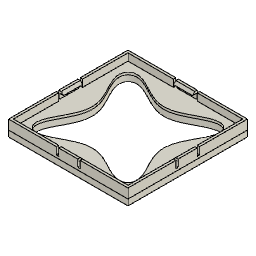
aufsatz (v3) v6 (Autodesk Fusion 360 design; units mm, degrees)
Autodesk Fusion 360 part; units mm, degrees
sketch "Skizze1" plane through (0, 0, 0) normal (0, 0, 1) x (1, 0, 0)
  line L0 (25, -25) -> (-25, -25) construction
  line L1 (-25, -25) -> (-25, 25) construction
  line L2 (-25, 25) -> (25, 25) construction
  line L3 (25, 25) -> (25, -25) construction
  line L4 (25, -25) -> (-25, 25) construction
  line L5 (-25, -25) -> (25, 25) construction
  line L6 (0, 25) -> (0, 20) construction
  line L7 (2.5, 22.5) -> (-2.5, 22.5)
  line L8 (-2.5, 22.5) -> (-2.5, 17.5)
  line L9 (-2.5, 17.5) -> (2.5, 17.5)
  line L10 (2.5, 17.5) -> (2.5, 22.5)
  line L11 (2.5, 22.5) -> (-2.5, 17.5) construction
  line L12 (-2.5, 22.5) -> (2.5, 17.5) construction
  circle A0 centre (0, 20) radius 5 construction
  line L13 (-22.5, -2.5) -> (-17.5, -2.5)
  line L14 (-17.5, -2.5) -> (-17.5, 2.5)
  line L15 (-22.5, 2.5) -> (-22.5, -2.5)
  line L16 (-17.5, 2.5) -> (-22.5, 2.5)
  line L17 (2.5, -22.5) -> (2.5, -17.5)
  line L18 (2.5, -17.5) -> (-2.5, -17.5)
  line L19 (-2.5, -22.5) -> (2.5, -22.5)
  line L20 (-2.5, -17.5) -> (-2.5, -22.5)
  line L21 (22.5, 2.5) -> (17.5, 2.5)
  line L22 (17.5, 2.5) -> (17.5, -2.5)
  line L23 (22.5, -2.5) -> (22.5, 2.5)
  line L24 (17.5, -2.5) -> (22.5, -2.5)
  line L25 (0, 25) -> (0, 15) construction
  line L26 (-25, -25) -> (25, -25)
  line L27 (25, -25) -> (25, 25)
  line L28 (25, 25) -> (-25, 25)
  line L29 (-25, 25) -> (-25, -25)
  spline S0 degree 5 poles (-20.0503, -20.0503) (-19.6556, -20.4489) (-18.686, -21.0653) (-16.7589, -21.3768) (-13.6473, -20.413) (-9.2487, -17.9258) (-4.6595, -15.5152) (0, -14.5056) (4.6595, -15.5149) (9.249, -17.9252) (13.6484, -20.4119) (17.5385, -21.6165) (20.5241, -20.5233) (21.5929, -17.5167) (20.3741, -13.6196) (17.8872, -9.2258) (15.4909, -4.649) (14.5051, -0.0015) (15.5403, 4.6523) (17.9692, 9.2426) (20.4589, 13.6458) (21.6478, 17.539) (20.5227, 20.524) (17.4867, 21.5928) (13.5795, 20.3782) (9.1932, 17.896) (4.6342, 15.5003) (0.0037, 14.5069) (-4.642, 15.5269) (-9.233, 17.9402) (-13.6414, 20.424) (-17.5392, 21.6225) (-20.5241, 20.5233) (-21.5922, 17.5107) (-20.3811, 13.6075) (-17.9032, 9.2107) (-15.5084, 4.637) (-14.5087, 0.0002) (-15.515, -4.6374) (-17.9137, -9.2128) (-20.3911, -13.611) (-21.3564, -16.7334) (-21.0536, -18.6733) (-20.4449, -19.6516) (-20.0503, -20.0503) knots 0 0 0 0 0 0 0.025 0.05 0.075 0.1 0.125 0.15 0.175 0.2 0.225 0.25 0.275 0.3 0.325 0.35 0.375 0.4 0.425 0.45 0.475 0.5 0.525 0.55 0.575 0.6 0.625 0.65 0.675 0.7 0.725 0.75 0.775 0.8 0.825 0.85 0.875 0.9 0.925 0.95 0.975 1 1 1 1 1 1
  line L30 (-15.1005, 25.0697) -> (-25, 15.0308)
  line L31 (25.1278, 15.1005) -> (14.9727, 25)
  line L32 (-25, -15.0497) -> (-15.1005, -25.0508)
  line L33 (15.1005, -25.0545) -> (25, -15.046)
  point P0 (0, 20)
  point P1 (0, -15)
  point P2 (20.0503, -20.0503)
  point P3 (15, 0)
  point P4 (20.0503, 20.0503)
  point P5 (-20.0503, 20.0503)
  point P6 (-15, 0)
  dimension "d1" = 50
  dimension "d2" = 50
  dimension "d3" = 5
  dimension "d4" = 5
  dimension "d5" = 5
  dimension "d7" = 10
  dimension "d14" = 10
  dimension "d19" = 7
  dimension "d20" = 7
  dimension "d21" = 7
  dimension "d22" = 7
  constraint horizontal L0
  constraint perpendicular L0 L1
  constraint parallel L0 L2
  constraint parallel L1 L3
  constraint coincident L4 origin
  constraint coincident L5 origin
  constraint midpoint L2 L6.start
  constraint perpendicular L2 L6
  constraint horizontal L7
  constraint perpendicular L7 L8
  constraint parallel L7 L9
  constraint parallel L8 L10
  constraint coincident L11 P0
  constraint coincident L12 P0
  constraint coincident P0 L6.end
  constraint coincident L6.start L25.start
  constraint parallel L6 L25
  constraint horizontal L26
  constraint vertical L27
  constraint horizontal L28
  constraint vertical L29
  constraint coincident L5 S0.start
  constraint coincident L4 P2
  constraint coincident L5 P4
  constraint coincident L4 P5
  constraint midpoint P5 L30
  constraint coincident L1 L30.end
  constraint midpoint P4 L31
  constraint coincident L28 L31.end
  constraint midpoint S0.start L32
  constraint midpoint P2 L33
  constraint coincident L3 L33.end
  measures "d1" distance of L1.end L2.end
  measures "d2" distance of L0.end L1.end
  measures "d3" distance of L6.start P0
  measures "d4" distance of L8.end L9.end
  measures "d5" distance of L7.end L8.end
  measures "d7" diameter of A0
  measures "d14" distance of L6.start L25.end
  measures "d19" distance of L1.end P5
  measures "d20" distance of L2.end P4
  measures "d21" distance of L0.start P2
  measures "d22" distance of L0.end S0.start
extrude "Extrusion6" add sketch "Skizze1" against normal blind 2.5 contours L26 L29 L32 | L26 S0 L32 L33 | L29 S0 L30 L32 | L26 L27 L33 | L28 L29 L30 | L27 S0 L31 L33 | L28 S0 L30 L31 | L27 L28 L31 makes body 1
extrude "Extrusion5" add sketch "Skizze1" along normal blind 1 separate body contours L7 L8 L9 L10 | L13 L14 L15 L16 | L17 L18 L19 L20 | L21 L22 L23 L24 | L26 L29 L32 | L26 S0 L32 L33 | L29 S0 L30 L32 | L26 L27 L33 | L28 L29 L30 | L27 S0 L31 L33 | L28 S0 L30 L31 | L27 L28 L31 makes body 2
sketch "Skizze4" plane through (0, 0, 1) normal (0, 0, 1) x (-1, 0, 0)
  spline S0 degree 5 poles (20.0503, 20.0503) (20.4449, 19.6516) (21.0536, 18.6733) (21.3564, 16.7334) (20.3911, 13.611) (17.9137, 9.2128) (15.515, 4.6374) (14.5087, -0.0002) (15.5084, -4.637) (17.9032, -9.2107) (20.3811, -13.6075) (21.5922, -17.5107) (20.5241, -20.5233) (17.5392, -21.6225) (13.6414, -20.424) (9.233, -17.9402) (4.642, -15.5269) (-0.0037, -14.5069) (-4.6342, -15.5003) (-9.1932, -17.896) (-13.5795, -20.3782) (-17.4867, -21.5928) (-20.5227, -20.524) (-21.6478, -17.539) (-20.4589, -13.6458) (-17.9692, -9.2426) (-15.5403, -4.6523) (-14.5051, 0.0015) (-15.4909, 4.649) (-17.8872, 9.2258) (-20.3741, 13.6196) (-21.5929, 17.5167) (-20.5241, 20.5233) (-17.5385, 21.6165) (-13.6484, 20.4119) (-9.249, 17.9252) (-4.6595, 15.5149) (0, 14.5056) (4.6595, 15.5152) (9.2487, 17.9258) (13.6473, 20.413) (16.7589, 21.3768) (18.686, 21.0653) (19.6556, 20.4489) (20.0503, 20.0503) knots -1 -1 -1 -1 -1 -1 -0.975 -0.95 -0.925 -0.9 -0.875 -0.85 -0.825 -0.8 -0.775 -0.75 -0.725 -0.7 -0.675 -0.65 -0.625 -0.6 -0.575 -0.55 -0.525 -0.5 -0.475 -0.45 -0.425 -0.4 -0.375 -0.35 -0.325 -0.3 -0.275 -0.25 -0.225 -0.2 -0.175 -0.15 -0.125 -0.1 -0.075 -0.05 -0.025 0 0 0 0 0 0
  line L0 (25, -25) -> (25, 25)
  line L1 (25, 25) -> (-25, 25)
  line L2 (-25, 25) -> (-25, -25)
  line L3 (-25, -25) -> (25, -25)
  line L4 (25, -5) -> (25, -25)
  line L5 (25, -25) -> (5, -25)
  line L6 (5, -25) -> (5, -24)
  line L7 (5, -24) -> (24, -24)
  line L8 (24, -24) -> (24, -5)
  line L9 (24, -5) -> (25, -5)
  line L10 (0, -25) -> (0, -15)
  line L11 (-5, -25) -> (-5, -24)
  line L12 (-5, -24) -> (-24, -24)
  line L13 (-24, -24) -> (-24, -5)
  line L14 (-24, -5) -> (-25, -5)
  line L15 (-25, -5) -> (-25, -25)
  line L16 (-25, -25) -> (-5, -25)
  line L17 (-25, 5) -> (-24, 5)
  line L18 (-24, 5) -> (-24, 24)
  line L19 (-24, 24) -> (-5, 24)
  line L20 (-5, 24) -> (-5, 25)
  line L21 (-5, 25) -> (-25, 25)
  line L22 (-25, 25) -> (-25, 5)
  line L23 (25, 5) -> (24, 5)
  line L24 (24, 5) -> (24, 24)
  line L25 (24, 24) -> (5, 24)
  line L26 (5, 24) -> (5, 25)
  line L27 (5, 25) -> (25, 25)
  line L28 (25, 25) -> (25, 5)
  line L29 (25, -4) -> (23, -4)
  line L30 (23, -4) -> (23, 4)
  line L31 (23, 4) -> (25, 4)
  line L32 (25, 4) -> (25, -4)
  line L33 (4, 25) -> (-4, 25)
  line L34 (-4, 25) -> (-4, 23)
  line L35 (-4, 23) -> (4, 23)
  line L36 (4, 23) -> (4, 25)
  line L37 (-25, -4) -> (-23, -4)
  line L38 (-23, -4) -> (-23, 4)
  line L39 (-23, 4) -> (-25, 4)
  line L40 (-25, 4) -> (-25, -4)
  line L41 (4, -25) -> (-4, -25)
  line L42 (-4, -25) -> (-4, -23)
  line L43 (-4, -23) -> (4, -23)
  line L44 (4, -23) -> (4, -25)
  point P0 (25, 0)
  point P1 (-25, 0)
  point P2 (0, 25)
  dimension "d38" = 1
  dimension "d39" = 1
  dimension "d40" = 5
  dimension "d41" = 5
  dimension "d44" = 1
  dimension "d45" = 1
  dimension "d46" = 1
  dimension "d47" = 1
  dimension "d48" = 1
  dimension "d49" = 1
  dimension "d50" = 5
  dimension "d51" = 10
  dimension "d52" = 5
  dimension "d53" = 5
  dimension "d54" = 5
  dimension "d55" = 5
  dimension "d56" = 2
  dimension "d57" = 1
  dimension "d60" = 1
  dimension "d61" = 1
  dimension "d62" = 1
  dimension "d63" = 2
  dimension "d64" = 2
  dimension "d65" = 1
  dimension "d66" = 1
  dimension "d67" = 2
  dimension "d68" = 1
  dimension "d69" = 1
  constraint coincident L0 L4.start
  constraint coincident L0.start L3.end
  constraint perpendicular L3 L4
  constraint coincident L3 L5.end
  constraint perpendicular L0 L5
  constraint perpendicular L3 L6
  constraint perpendicular L0 L7
  constraint perpendicular L3 L8
  constraint midpoint L0 P0
  constraint coincident L3 L11.start
  constraint perpendicular L3 L11
  constraint perpendicular L11 L12
  constraint perpendicular L3 L13
  constraint coincident L2 L14.end
  constraint perpendicular L2 L14
  constraint coincident L2.end L3.start
  constraint perpendicular L3 L15
  constraint coincident L2 L17.start
  constraint perpendicular L2 L17
  constraint perpendicular L1 L18
  constraint perpendicular L18 L19
  constraint coincident L1 L20.end
  constraint perpendicular L1 L20
  constraint coincident L1.end L2.start
  constraint perpendicular L2 L21
  constraint perpendicular L1 L22
  constraint coincident L0 L23.start
  constraint perpendicular L0 L23
  constraint perpendicular L23 L24
  constraint perpendicular L24 L25
  constraint coincident L1 L26.end
  constraint perpendicular L1 L26
  constraint coincident L0.end L1.start
  constraint perpendicular L0 L27
  constraint midpoint L2 P1
  constraint midpoint L1 P2
  constraint horizontal L29
  constraint vertical L30
  constraint horizontal L31
  constraint vertical L32
  constraint coincident L0 L29.start
  constraint horizontal L9
  constraint horizontal L33
  constraint vertical L34
  constraint horizontal L35
  constraint vertical L36
  constraint coincident L1 L33.start
  constraint horizontal L37
  constraint vertical L38
  constraint horizontal L39
  constraint vertical L40
  constraint coincident L2 L37.start
  constraint horizontal L41
  constraint vertical L42
  constraint horizontal L43
  constraint vertical L44
  constraint coincident L3 L41.start
  measures "d38" distance of L4.start L8.end
  measures "d39" distance of L5.end L6.end
  measures "d40" distance of L6 L10
  measures "d41" distance of L9 P0
  measures "d44" distance of L18 L22
  measures "d45" distance of L19 L21
  measures "d46" distance of L25 L27
  measures "d47" distance of L24 L28
  measures "d48" distance of L13 L15
  measures "d49" distance of L12 L16
  measures "d50" distance of L10.start L11
  measures "d51" distance of L14 L17
  measures "d52" distance of L17.start P1
  measures "d53" distance of P0 L23.start
  measures "d54" distance of L26.end P2
  measures "d55" distance of L20.end P2
  measures "d56" distance of L30.end L31.end
  measures "d57" distance of L23 L31
  measures "d60" distance of L9 L29
  measures "d61" distance of L26 L36
  measures "d62" distance of L20 L34
  measures "d63" distance of L33.end L34.end
  measures "d64" distance of L37.start L37.end
  measures "d65" distance of L14 L37
  measures "d66" distance of L17 L39
  measures "d67" distance of L41.start L43.end
  measures "d68" distance of L6 L44
  measures "d69" distance of L11 L42
extrude "Extrusion8" add sketch "Skizze4" along normal blind 3 contours L0 L3 L4 L5 L6 L7 L8 L9 | L0 L29 L30 L31 L32 | L3 L10 L41 L43 L44 | L3 L10 L41 L42 L43 | L0 L1 L23 L24 L25 L26 L27 L28 | L2 L3 L11 L12 L13 L14 L15 L16 | L1 L33 L34 L35 L36 | L2 L37 L38 L39 L40 | L1 L2 L17 L18 L19 L20 L21 L22 bodies 2
extrude "Extrusion7" add sketch "Skizze4" along normal blind 2 contours L0 L3 L4 L5 L6 L7 L8 L9 bodies 2
sketch "Skizze5" plane through (4, 0, 0) normal (1, 0, 0) x (0, 1, 0)
  line L0 (23, 1) -> (25, 1)
  line L1 (25, 1) -> (25, 4)
  line L2 (25, 4) -> (23, 4)
  line L3 (23, 4) -> (23, 1)
  line L4 (23, 1) -> (24.5, 1)
  line L5 (24.5, 1) -> (24.5, 3)
  line L6 (24.5, 3) -> (23, 3)
  line L7 (23, 3) -> (23, 1)
  line L8 (23, 3) -> (24, 4)
  line L9 (24, 4) -> (23, 4)
  line L10 (23, 4) -> (23, 3)
  dimension "d72" = 1.5
  dimension "d73" = 2
  constraint horizontal L4
  constraint vertical L5
  constraint horizontal L6
  constraint vertical L7
  constraint coincident L0.start L3.end
  constraint midpoint L2 L8.end
  constraint coincident L2.end L3.start
  measures "d72" distance of L5.end L6.end
  measures "d73" distance of L4.end L5.end
extrude "Extrusion9" cut sketch "Skizze5" against normal blind 8 contours L0 L3 L4 L5 L6 L7 | L2 L3 L8 L9 L10 bodies 2
sketch "Skizze6" plane through (0, -4, 0) normal (0, -1, 0) x (1, 0, 0)
  line L0 (-25, 1) -> (-23, 1)
  line L1 (-23, 1) -> (-23, 4)
  line L2 (-23, 4) -> (-25, 4)
  line L3 (-25, 4) -> (-25, 1)
  line L4 (-23, 1) -> (-24.5, 1)
  line L5 (-24.5, 1) -> (-24.5, 3)
  line L6 (-24.5, 3) -> (-23, 3)
  line L7 (-23, 3) -> (-23, 1)
  line L8 (-23, 3) -> (-24, 4)
  line L9 (-24, 4) -> (-24, 3)
  constraint horizontal L4
  constraint vertical L5
  constraint horizontal L6
  constraint vertical L7
  constraint coincident L0.end L1.start
  constraint midpoint L2 L8.end
  constraint coincident L6 L9.end
  constraint perpendicular L6 L9
extrude "Extrusion10" cut sketch "Skizze6" against normal blind 8 contours L0 L1 L4 L5 L6 L7 | L1 L2 L8 bodies 2
sketch "Skizze7" plane through (4, 0, 0) normal (1, 0, 0) x (0, 1, 0)
  line L0 (-25, 1) -> (-23, 1)
  line L1 (-23, 1) -> (-23, 4)
  line L2 (-23, 4) -> (-25, 4)
  line L3 (-25, 4) -> (-25, 1)
  line L4 (-23, 1) -> (-24.5, 1)
  line L5 (-24.5, 1) -> (-24.5, 3)
  line L6 (-24.5, 3) -> (-23, 3)
  line L7 (-23, 3) -> (-23, 1)
  line L8 (-23, 3) -> (-24, 4)
  line L9 (-24, 3) -> (-24, 4)
  constraint horizontal L4
  constraint vertical L5
  constraint horizontal L6
  constraint vertical L7
  constraint coincident L0.end L1.start
  constraint midpoint L2 L8.end
  constraint coincident L6 L9.start
extrude "Extrusion11" cut sketch "Skizze7" against normal blind 8 contours L0 L1 L4 L5 L6 L7 | L1 L2 L8 bodies 2
sketch "Skizze8" plane through (0, -4, 0) normal (0, -1, 0) x (1, 0, 0)
  line L0 (23, 1) -> (25, 1)
  line L1 (25, 1) -> (25, 4)
  line L2 (25, 4) -> (23, 4)
  line L3 (23, 4) -> (23, 1)
  line L4 (23, 1) -> (24.5, 1)
  line L5 (24.5, 1) -> (24.5, 3)
  line L6 (24.5, 3) -> (23, 3)
  line L7 (23, 3) -> (23, 1)
  line L8 (23, 3) -> (24, 4)
  line L9 (24, 4) -> (24, 3)
  constraint horizontal L4
  constraint vertical L5
  constraint horizontal L6
  constraint vertical L7
  constraint coincident L0.start L3.end
  constraint midpoint L2 L8.end
  constraint coincident L6 L9.end
  constraint perpendicular L6 L9
extrude "Extrusion12" cut sketch "Skizze8" against normal blind 8 contours L0 L3 L4 L5 L6 L7 | L2 L3 L8 bodies 2
